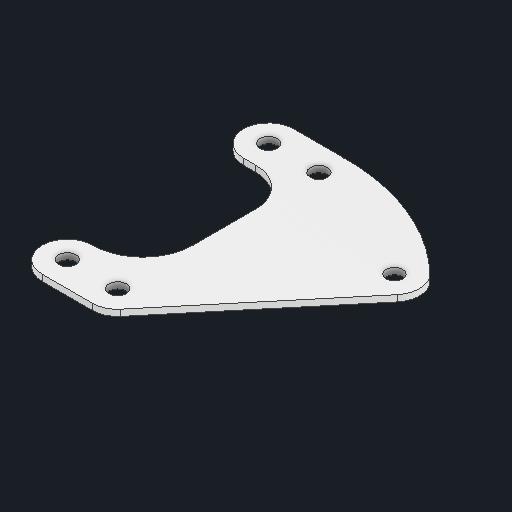
# Autodesk Inventor part: gusset
Saved by Autodesk Inventor 2025 (Build 290162000, 162)
## iProperties
Created: 2024-08-21
Part Number: gusset
Material: Acetal Resin, White
Document SubType Name: Sheet Metal
Designer: averey
Density: 1.425 g/cm^3
Appearance: Smooth - White
Flat Pattern Width: 5.49906 cm
Flat Pattern Length: 7.05463 cm
Flat Pattern Area: 38.7938 cm^2
Sheet Metal Rule: Default_mm
Sheet Metal Width: 2.165 in
Sheet Metal Length: 2.777 in
Sheet Metal Area: 6.013 in^2
d0: 0.500 in
d1: 0.500 in
d2: 0.375 in
Author: averey
Autodesk Inventor part; units mm, degrees
ref_plane "YZ Plane" through (0, 0, 0) normal (1, 0, 0) x (0, 1, 0)
ref_plane "XZ Plane" through (0, 0, 0) normal (0, 1, 0) x (-1, 0, 0)
ref_plane "XY Plane" through (0, 0, 0) normal (0, 0, 1) x (1, 0, 0)
sketch "main" plane through (0, 0, 0) normal (0, 0, 1) x (1, 0, 0)
  arc A0 (24.1925, 23.7791) -> (11.4925, 11.0791) centre (24.1925, 11.0791) ccw
  circle A1 centre (11.4925, 30.1291) radius 2.1844
  line L0 (24.1925, 23.7791) -> (24.1925, 23.7791)
  arc A2 (11.4925, 36.4791) -> (6.6143, 34.1942) centre (11.4925, 30.1291) ccw
  circle A3 centre (24.1925, 30.1291) radius 2.1844
  line L1 (24.1925, 36.4791) -> (11.4925, 36.4791)
  arc A4 (24.1925, 23.7791) -> (24.1925, 36.4791) centre (24.1925, 30.1291) ccw
  circle A5 centre (11.4925, -20.6709) radius 2.1844
  circle A6 centre (24.1925, -20.6709) radius 2.1844
  line L2 (24.1925, -14.3081) -> (21.0175, -14.3081)
  arc A7 (24.1539, -27.0337) -> (24.1925, -14.3081) centre (24.1925, -20.6709) ccw
  line L3 (11.4925, 11.0791) -> (11.4925, -4.7831)
  line L4 (6.6143, 34.1942) -> (-25.1357, -3.9059)
  arc A8 (11.4925, -4.7831) -> (21.0175, -14.3081) centre (21.0175, -4.7831) ccw
  circle A9 centre (-20.2575, -7.971) radius 2.0955
  arc A10 (-24.6678, -12.5396) -> (11.5311, -27.0337) centre (11.2178, 24.6342) ccw
  arc A11 (-25.1357, -3.9059) -> (-24.6678, -12.5396) centre (-20.2575, -7.971) ccw
  line L5 (11.5311, -27.0337) -> (24.2311, -27.0337)
  point P0 (10.6662, 5.6616)
  point P1 (11.4925, 23.7791)
  point P2 (11.4925, -14.3081)
  dimension "d0" = 12.7
  dimension "d1" = 12.7
  dimension "d2" = 9.525
  measures "d0" diameter of A11
  measures "d1" radius of A0
  measures "d2" radius of A8
sketch "Sketch1" plane through (0, 0, 0) normal (0, 1, 0) x (-1, 0, 0)
  arc A0 (24.1925, 23.7791) -> (11.4925, 11.0791) centre (24.1925, 11.0791) ccw
  circle A1 centre (11.4925, 30.1291) radius 2.1844
  line L0 (24.1925, 23.7791) -> (24.1925, 23.7791)
  arc A2 (11.4925, 36.4791) -> (6.6143, 34.1942) centre (11.4925, 30.1291) ccw
  circle A3 centre (24.1925, 30.1291) radius 2.1844
  line L1 (24.1925, 36.4791) -> (11.4925, 36.4791)
  arc A4 (24.1925, 23.7791) -> (24.1925, 36.4791) centre (24.1925, 30.1291) ccw
  circle A5 centre (11.4925, -20.6709) radius 2.1844
  circle A6 centre (24.1925, -20.6709) radius 2.1844
  line L2 (24.1925, -14.3081) -> (21.0175, -14.3081)
  arc A7 (24.1539, -27.0337) -> (24.1925, -14.3081) centre (24.1925, -20.6709) ccw
  line L3 (11.4925, 11.0791) -> (11.4925, -4.7831)
  line L4 (6.6143, 34.1942) -> (-25.1357, -3.9059)
  arc A8 (11.4925, -4.7831) -> (21.0175, -14.3081) centre (21.0175, -4.7831) ccw
  circle A9 centre (-20.2575, -7.971) radius 2.0955
  arc A10 (-24.6678, -12.5396) -> (11.5311, -27.0337) centre (11.2178, 24.6342) ccw
  arc A11 (-25.1357, -3.9059) -> (-24.6678, -12.5396) centre (-20.2575, -7.971) ccw
  line L5 (11.5311, -27.0337) -> (24.2311, -27.0337)
  point P0 (0, 0)
extrude "Extrusion1" add sketch "Sketch1" along normal blind 1.5875
equation "\"BendRadius\" = Thickness"
equation "\"BendReliefWidth\" = Thickness"
equation "\"BendReliefDepth\" = 0.5 * Thickness"
equation "\"CornerReliefSize\" = 4 * Thickness"
equation "\"MinimumRemnant\" = 2 * Thickness"
equation "\"TransitionRadius\" = BendRadius"
equation "\"JacobiRadiusSize\" = BendRadius"
equation "\"GapSize\" = Thickness"
equation "\"Thickness\" = 1.5875"
body "Solid1"
